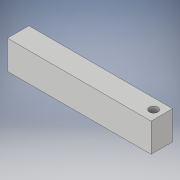
# Autodesk Inventor part: Side Bar
Saved by Autodesk Inventor 2017 (Build 210142000, 142)
## iProperties
Created: 2017-10-11
Part Number: Side Bar
Material: Generic
Document SubType Name: Modeling
Designer: Kenneth
Density: 1 g/cm^3
Appearance: Default
Author: Kenneth
Autodesk Inventor part; units mm, degrees
ref_plane "YZ Plane" through (0, 0, 0) normal (1, 0, 0) x (0, 1, 0)
ref_plane "XZ Plane" through (0, 0, 0) normal (0, 1, 0) x (-1, 0, 0)
ref_plane "XY Plane" through (0, 0, 0) normal (0, 0, 1) x (1, 0, 0)
sketch "Sketch1" plane through (0, 0, 0) normal (0, 0, 1) x (1, 0, 0)
  line L0 (-63.5, -12.7) -> (63.5, -12.7)
  line L1 (63.5, -12.7) -> (63.5, 12.7)
  line L2 (63.5, 12.7) -> (-63.5, 12.7)
  line L3 (-63.5, 12.7) -> (-63.5, -12.7)
  line L4 (-63.5, -12.7) -> (63.5, 12.7) construction
  line L5 (63.5, -12.7) -> (-63.5, 12.7) construction
  point P0 (0, 0)
  dimension "d0" = 127
  dimension "d1" = 25.4
  constraints: 12 end point, 2 midpoint, 2 parallel, 1 horizontal, 1 perpendicular
  measures "d0" distance of L1.end L2.end
  measures "d1" distance of L0.end L1.end
extrude "Extrusion1" add sketch "Sketch1" along normal blind 19.05
sketch "Sketch3" plane through (-63.5, 12.7, 0) normal (0, 1, 0) x (1, 0, 0)
  circle A0 centre (119.38, -9.1052) radius 3.81
  line L0 (0, 0) -> (0, -19.05) projected
  line L1 (127, 0) -> (127, -19.05) projected
  point P0 (63.5, 0)
  dimension "d12" = 7.62
  dimension "d14" = 7.62
  constraints: 1 centre point
  measures "d12" diameter of A0
  measures "d14" distance from line of L1 A0.centre
extrude "Extrusion3" cut sketch "Sketch3" against normal blind 25.4
body "Solid1"
